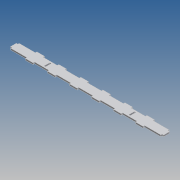
# Autodesk Inventor part: CaissonArriere
Saved by Autodesk Inventor 2019 (Build 230136000, 136)
## iProperties
Created: 2019-08-26
Part Number: CaissonArriere
Material: PVC-U
Document SubType Name: Modeling
Designer: jeremias.salamin
Density: 1.4 g/cm^3
Appearance: Lisse - Blanc
Description: CaissonArrière
Mass: 3.09084 g
Surface Area: 32.896 cm^2
Volume: 2.20774 cm^3
Author: jeremias.salamin
Autodesk Inventor part; units mm, degrees
ref_plane "YZ Plane" through (0, 0, 0) normal (1, 0, 0) x (0, 1, 0)
ref_plane "XZ Plane" through (0, 0, 0) normal (0, 1, 0) x (-1, 0, 0)
ref_plane "XY Plane" through (0, 0, 0) normal (0, 0, 1) x (1, 0, 0)
sketch "Sketch1" plane through (0, 0, 0) normal (0, 0, 1) x (1, 0, 0)
  line L0 (0, 6.16) -> (0, -6.16) construction
  line L1 (-109.76, 0) -> (109.76, 0) construction
  line L2 (78.4, -4.4) -> (-78.4, -4.4)
  line L3 (-78.4, -4.4) -> (-78.4, 4.4)
  line L4 (-78.4, 4.4) -> (78.4, 4.4)
  line L5 (78.4, 4.4) -> (78.4, -4.4)
  line L6 (78.4, -4.4) -> (-78.4, 4.4) construction
  line L7 (-78.4, -4.4) -> (78.4, 4.4) construction
  point P0 (0, 0)
  dimension "d0" = 156.8
  dimension "d1" = 8.8
  constraints: 12 end point, 2 midpoint, 2 parallel, 1 horizontal, 1 perpendicular
  measures "d0" distance of L3.end L4.end
  measures "d1" distance of L2.end L3.end
extrude "Extrusion1" add sketch "Sketch1" along normal mid plane 1.6
sketch "Esquisse3" plane through (0, 0, 0.8) normal (0, 0, 1) x (1, 0, 0)
  line L0 (-78.4, -4.4) -> (78.4, -4.4) construction
  line L1 (78.4, -4.4) -> (78.4, 4.4) construction
  line L2 (78.4, 4.4) -> (-78.4, 4.4) construction
  line L3 (-78.4, 4.4) -> (-78.4, -4.4) construction
  line L4 (-112, 0) -> (112, 0) construction
  line L5 (0, 8.08) -> (0, -6.48) construction
  line L6 (-78.4, 3) -> (-80, 3)
  line L7 (-80, 3) -> (-80, -3)
  line L8 (-80, -3) -> (-78.4, -3)
  line L9 (-78.4, -3) -> (-78.4, 3)
  line L10 (78.4, 3) -> (80, 3)
  line L11 (80, 3) -> (80, -3)
  line L12 (80, -3) -> (78.4, -3)
  line L13 (78.4, -3) -> (78.4, 3)
  point P0 (0, 0)
  dimension "d15" = 1.6
  dimension "d16" = 6
  constraints: 16 end point, 4 symmetric about line, 2 parallel, 1 horizontal, 1 perpendicular, 1 point on line, 1 other
  measures "d15" distance of L8.end L7.end
  measures "d16" distance of L7.end L6.end
extrude "Extrusion3" add sketch "Esquisse3" against normal blind 1.6
sketch "Esquisse4" plane through (0, 0, 0.8) normal (0, 0, 1) x (1, 0, 0)
  line L0 (80, 3) -> (80, -3) construction
  line L1 (80, -3) -> (78.4, -3) construction
  line L2 (78.4, -3) -> (78.4, -4.4) construction
  line L3 (78.4, -4.4) -> (-78.4, -4.4) construction
  line L4 (-78.4, -4.4) -> (-78.4, -3) construction
  line L5 (-78.4, -3) -> (-80, -3) construction
  line L6 (-80, -3) -> (-80, 3) construction
  line L7 (-80, 3) -> (-78.4, 3) construction
  line L8 (-78.4, 3) -> (-78.4, 4.4) construction
  line L9 (-78.4, 4.4) -> (78.4, 4.4) construction
  line L10 (78.4, 4.4) -> (78.4, 3) construction
  line L11 (78.4, 3) -> (80, 3) construction
  line L12 (-78.4, -4.4) -> (78.4, -4.4) construction
  line L13 (78.4, -4.4) -> (78.4, -3) construction
  line L14 (78.4, -3) -> (80, -3) construction
  line L15 (80, -3) -> (80, 3) construction
  line L16 (80, 3) -> (78.4, 3) construction
  line L17 (78.4, 3) -> (78.4, 4.4) construction
  line L18 (78.4, 4.4) -> (-78.4, 4.4) construction
  line L19 (-78.4, 4.4) -> (-78.4, 3) construction
  line L20 (-78.4, 3) -> (-80, 3) construction
  line L21 (-80, 3) -> (-80, -3) construction
  line L22 (-80, -3) -> (-78.4, -3) construction
  line L23 (-78.4, -3) -> (-78.4, -4.4) construction
  line L24 (0, 8.08) -> (0, -6.48) construction
  line L25 (-112, 0) -> (112, 0) construction
  line L26 (-61.5, 4.4) -> (-53.5, 4.4)
  line L27 (-53.5, 4.4) -> (-53.5, 6)
  line L28 (-53.5, 6) -> (-61.5, 6)
  line L29 (-61.5, 6) -> (-61.5, 4.4)
  line L30 (-30.5, 4.4) -> (-30.5, 6)
  line L31 (-38.5, 4.4) -> (-30.5, 4.4)
  line L32 (-30.5, 6) -> (-38.5, 6)
  line L33 (-38.5, 6) -> (-38.5, 4.4)
  line L34 (-7.5, 4.4) -> (-7.5, 6)
  line L35 (-15.5, 4.4) -> (-7.5, 4.4)
  line L36 (-7.5, 6) -> (-15.5, 6)
  line L37 (-15.5, 6) -> (-15.5, 4.4)
  line L38 (15.5, 4.4) -> (15.5, 6)
  line L39 (7.5, 4.4) -> (15.5, 4.4)
  line L40 (15.5, 6) -> (7.5, 6)
  line L41 (7.5, 6) -> (7.5, 4.4)
  line L42 (38.5, 4.4) -> (38.5, 6)
  line L43 (30.5, 4.4) -> (38.5, 4.4)
  line L44 (38.5, 6) -> (30.5, 6)
  line L45 (30.5, 6) -> (30.5, 4.4)
  line L46 (61.5, 4.4) -> (61.5, 6)
  line L47 (53.5, 4.4) -> (61.5, 4.4)
  line L48 (61.5, 6) -> (53.5, 6)
  line L49 (53.5, 6) -> (53.5, 4.4)
  point P0 (0, 0)
  dimension "d19" = 8
  dimension "d20" = 1.6
  dimension "d23" = 23
  constraints: 48 end point, 2 horizontal, 2 parallel, 1 perpendicular, 1 point on line, 41 other
  measures "d19" distance of L28.end L27.end
  measures "d20" distance of L27.end L26.end
  measures "d23" distance of L26.end L30.start
extrude "Extrusion4" add sketch "Esquisse4" against normal blind 1.6
mirror "Symétrie2" about plane through (0, 0, 0) normal (0, 1, 0) of "Extrusion4"
sketch "Esquisse5" plane through (0, 0, 0.8) normal (0, 0, 1) x (1, 0, 0)
  line L0 (45, -3) -> (43.4, -3)
  line L1 (43.4, -3) -> (43.4, 3)
  line L2 (43.4, 3) -> (45, 3)
  line L3 (45, 3) -> (45, -3)
  line L4 (-43.4, -3) -> (-45, -3)
  line L5 (-45, -3) -> (-45, 3)
  line L6 (-45, 3) -> (-43.4, 3)
  line L7 (-43.4, 3) -> (-43.4, -3)
  point P0 (0, 0)
  constraints: 16 end point, 4 horizontal, 4 vertical, 8 other
extrude "Extrusion5" cut sketch "Esquisse5" against normal blind 1.6
